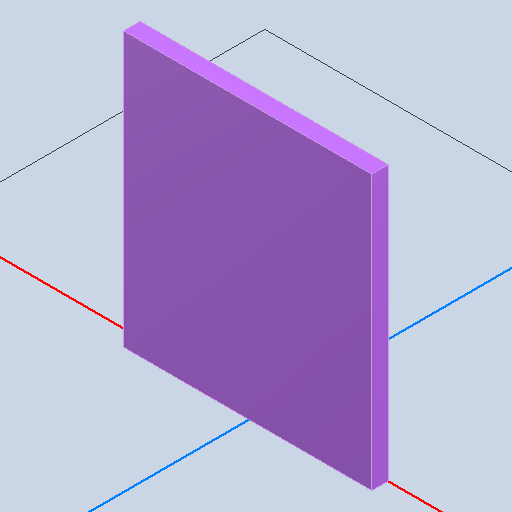
# Autodesk Inventor part: LMZ13610
Saved by Autodesk Inventor 2022 (Build 260153000, 153)
## iProperties
Created: 2022-02-26
Part Number: LMZ13610
Material: Типовые
Document SubType Name: Modeling
Designer: Petrov Ivan
Density: 1 g/cm^3
Appearance: LMZ13610, LMZ13610
Author: Petrov Ivan
Autodesk Inventor part; units mm, degrees
ref_plane "YZ Plane" through (0, 0, 0) normal (1, 0, 0) x (0, 1, 0)
ref_plane "XZ Plane" through (0, 0, 0) normal (0, 1, 0) x (-1, 0, 0)
ref_plane "XY Plane" through (0, 0, 0) normal (0, 0, 1) x (1, 0, 0)
sketch "LMZ13610, LMZ13610_27" plane through (0, 0, 0) normal (0, 0, 1) x (1, 0, 0)
  line L0 (-7.5635, 17.8435) -> (7.5, 17.8435)
  line L1 (7.5, 17.8435) -> (7.5, 1.2065)
  line L2 (7.5, 1.2065) -> (-7.5635, 1.2065)
  line L3 (-7.5635, 1.2065) -> (-7.5635, 17.8435)
  constraints: 8 end point
extrude "Выдавливание1" add sketch "LMZ13610, LMZ13610_27" along normal blind 1
